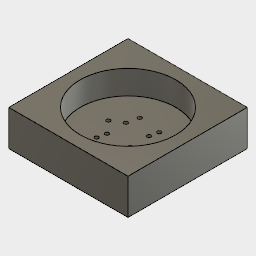
TreadForm v3 (Autodesk Fusion 360 design; units mm, degrees)
Autodesk Fusion 360 part; units mm, degrees
sketch "Sketch1" plane through (0, 0, 0) normal (0, 1, 0) x (1, 0, 0)
  line L0 (-63.5, 63.5) -> (63.5, 63.5)
  line L1 (63.5, 63.5) -> (63.5, -63.5)
  line L2 (63.5, -63.5) -> (-63.5, -63.5)
  line L3 (-63.5, -63.5) -> (-63.5, 63.5)
  constraint horizontal L0
  constraint vertical L1
  constraint horizontal L2
  constraint vertical L3
extrude "Extrude1" add sketch "Sketch1" along normal blind 38.1
sketch "Sketch2" plane through (0, 38.1, 0) normal (0, 1, 0) x (-1, 0, 0)
  line L0 (63.5, 63.5) -> (-63.5, 63.5)
  line L1 (-63.5, 63.5) -> (-63.5, -63.5)
  line L2 (-63.5, -63.5) -> (63.5, -63.5)
  line L3 (63.5, -63.5) -> (63.5, 63.5)
  circle A0 centre (0, 0) radius 50.8
  constraint coincident A0.centre origin
extrude "Extrude2" cut sketch "Sketch2" against normal blind 25.4 contours A0
sketch "Sketch6" plane through (0, 0, 0) normal (0, 1, 0) x (1, 0, 0)
  line L0 (-139.6725, 0.0069) -> (-172.6925, 0.0069)
  line L1 (-172.6925, -25.3931) -> (-139.6725, -25.3931)
  line L2 (-139.6725, -25.3931) -> (-139.6725, 0.0069)
  line L3 (-172.6925, -7.6131) -> (-177.7725, -7.6131)
  line L4 (-177.7725, -7.6131) -> (-177.7725, -5.0731)
  line L5 (-177.7725, -5.0731) -> (-182.8525, -5.0731)
  line L6 (-182.8525, -5.0731) -> (-182.8525, -20.3131)
  line L7 (-182.8525, -20.3131) -> (-177.7725, -20.3131)
  line L8 (-177.7725, -20.3131) -> (-177.7725, -17.7731)
  line L9 (-177.7725, -17.7731) -> (-172.6925, -17.7731)
  line L10 (-172.6925, 0.0069) -> (-172.6925, -7.6131)
  line L11 (-172.6925, -17.7731) -> (-172.6925, -25.3931)
  constraint horizontal L0
  constraint vertical L10
  constraint horizontal L1
  constraint vertical L2
  constraint perpendicular L3 L10
  constraint perpendicular L3 L4
  constraint perpendicular L4 L5
  constraint perpendicular L5 L6
  constraint perpendicular L6 L7
  constraint perpendicular L7 L8
  constraint perpendicular L8 L9
  constraint collinear L10 L11
sketch "Sketch9" plane through (0, 12.7, 0) normal (0, 1, 0) x (-1, 0, 0)
  circle A0 centre (0, 0) radius 50.8
  circle A1 centre (0, 0) radius 23.8125
  dimension "d23" = 47.625
  dimension "d24" = 60
  dimension "d25" = 60
  dimension "d26" = 60
  dimension "d27" = 60
  dimension "d28" = 60
  dimension "d29" = 60
  constraint concentric A0 A1
  constraint coincident A1
  constraint coincident A1 A0.centre
  measures "d23" diameter of A1
  measures "d24" angle of A0.centre
  measures "d27" angle of A0.centre
hole "Hole2" at (-23.6501, 12.7, -2.7764) at (-9.4206, 12.7, -21.8698) at (14.2295, 12.7, -19.0934) at (23.6501, 12.7, 2.7764) at (9.4206, 12.7, 21.8698) at (-14.2295, 12.7, 19.0934) direction (0, -1, 0) diameter 4.064 depth 50.8 tip angle 118
sketch "Sketch10" plane through (0, 12.7, 0) normal (0, 1, 0) x (-1, 0, 0)
  circle A0 centre (-9.4206, 21.8698) radius 2.032
  circle A1 centre (-14.2295, -19.0934) radius 2.032
  circle A2 centre (23.6501, -2.7764) radius 2.032
  circle A3 centre (9.4206, -21.8698) radius 2.032
  circle A4 centre (-23.6501, 2.7764) radius 2.032
  circle A5 centre (14.2295, 19.0934) radius 2.032
  circle A6 centre (0, 0) radius 50.8
  circle A7 centre (0, 0) radius 15.875
  dimension "d33" = 31.75
  constraint concentric A6 A7
  constraint coincident A7 A6.centre
  measures "d33" diameter of A7
hole "Hole3" at (-12.2777, 12.7, -10.0635) at (12.2777, 12.7, -10.0635) at (12.2777, 12.7, 10.0635) at (-12.2777, 12.7, 10.0635) direction (0, -1, 0) diameter 4.064 depth 50.8 tip angle 118
